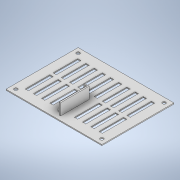
# Autodesk Inventor part: platforma
Saved by Autodesk Inventor 2020.3 (Build 243373000, 373)
## iProperties
Created: 2021-02-15
Part Number: platforma
Material: Ogólny
Document SubType Name: Modeling
Designer: sitar
Density: 1 g/cm^3
Appearance: Domyślna
Author: sitar
Autodesk Inventor part; units mm, degrees
ref_plane "YZ Plane" through (0, 0, 0) normal (1, 0, 0) x (0, 1, 0)
ref_plane "XZ Plane" through (0, 0, 0) normal (0, 1, 0) x (-1, 0, 0)
ref_plane "XY Plane" through (0, 0, 0) normal (0, 0, 1) x (1, 0, 0)
sketch "Szkic1" plane through (0, 0, 0) normal (0, 1, 0) x (-1, 0, 0)
  line L0 (58.5, -44) -> (-58.5, -44)
  line L1 (-58.5, -44) -> (-58.5, 44)
  line L2 (-58.5, 44) -> (58.5, 44)
  line L3 (58.5, 44) -> (58.5, -44)
  line L4 (58.5, -44) -> (-58.5, 44) construction
  line L5 (-58.5, -44) -> (58.5, 44) construction
  point P0 (0, 0)
  dimension "d0" = 117
  dimension "d1" = 88
  constraints: 12 end point, 2 midpoint, 2 parallel, 1 horizontal, 1 perpendicular
  measures "d0" distance of L1.end L2.end
  measures "d1" distance of L0.end L1.end
extrude "Wyciągnięcie proste1" add sketch "Szkic1" along normal blind 1.2
sketch "Szkic2" plane through (0, 1.2, 0) normal (0, 1, 0) x (1, 0, 0)
  line L0 (-52.5, 38) -> (-52.5, 44)
  line L1 (58.5, 44) -> (-58.5, 44) projected
  line L2 (-52.5, 38) -> (-46.5, 38) construction
  line L3 (-52.5, 38) -> (-58.5, 38)
  line L4 (-58.5, 44) -> (-58.5, -44) projected
  line L5 (-52.5, 38) -> (-46.5, 38) construction
  circle A0 centre (-52.5, 38) radius 2
  point P0 (0, 0)
  dimension "d4" = 6
  dimension "d5" = 90
  dimension "d6" = 6
  dimension "d7" = 180
  dimension "d8" = 4
  constraints: 8 end point, 2 equal length, 2 horizontal, 2 perpendicular, 2 point on line, 1 centre point, 1 coincident
  measures "d4" distance of L0.start L0.end
  measures "d5" angle of L2 L0
  measures "d6" distance of L0.start L3.end
  measures "d7" angle of L3 L5
  measures "d8" diameter of A0
extrude "Wyciągnięcie proste2" cut sketch "Szkic2" against normal through all contours L3 A0 L0 | L0 A0 L3
mirror "Odbij1" about plane through (0, 0, 0) normal (0, 0, 1) of "Wyciągnięcie proste2"
mirror "Odbij2" about plane through (0, 0, 0) normal (1, 0, 0) of "Wyciągnięcie proste2", "Odbij1"
sketch "Szkic3" plane through (0, 1.2, 0) normal (0, 1, 0) x (1, 0, 0)
  line L0 (-2.5, -34) -> (-58.5, -34)
  line L1 (-2.5, -34) -> (53.5, -34) construction
  line L2 (-2.5, -34) -> (-2.5, -44)
  line L3 (-2.5, -34) -> (7.5, -34) construction
  line L4 (-58.5, 44) -> (-58.5, -44) projected
  line L5 (-58.5, -44) -> (58.5, -44) projected
  circle A0 centre (-2.5, -34) radius 2
  line L6 (-2.5, -34) -> (-2.5, -12)
  line L7 (-2.5, -34) -> (19.5, -34) construction
  circle A1 centre (-2.5, -12) radius 2
  point P0 (0, 0)
  dimension "d11" = 56
  dimension "d12" = 180
  dimension "d13" = 10
  dimension "d14" = 90
  dimension "d15" = 4
  dimension "d16" = 22
  dimension "d17" = 90
  dimension "d18" = 4
  constraints: 12 end point, 4 horizontal, 3 equal length, 2 centre point, 2 coincident, 2 point on line, 2 vertical
  measures "d11" distance of L0.start L0.end
  measures "d12" angle of L0 L1
  measures "d13" distance of L0.start L2.end
  measures "d14" angle of L2 L3
  measures "d15" diameter of A0
  measures "d16" distance of L6.start L6.end
  measures "d17" angle of L7 L6
  measures "d18" diameter of A1
extrude "Wyciągnięcie proste3" add sketch "Szkic3" along normal blind 2 contours L2 A0 L0 | L6 A0 L2 | L0 A0 L6 | A1
sketch "Szkic4" plane through (-2.5, 3.2, 34) normal (0, 1, 0) x (1, 0, 0)
  circle A0 centre (0, 0) radius 1
  circle A1 centre (0, 22) radius 2 projected
  circle A2 centre (0, 22) radius 1
  point P0 (2.5, 34)
  dimension "d21" = 2
  dimension "d22" = 2
  constraints: 2 centre point, 1 coincident
  measures "d21" diameter of A0
  measures "d22" diameter of A2
extrude "Wyciągnięcie proste4" add sketch "Szkic4" along normal blind 4 contours A0 | A2
sketch "Szkic5" plane through (0, 1.2, 0) normal (0, 1, 0) x (1, 0, 0)
  line L0 (1.5, -4) -> (3.1, -4)
  line L1 (3.1, -4) -> (3.1, -39)
  line L2 (3.1, -39) -> (1.5, -39)
  line L3 (1.5, -39) -> (1.5, -4)
  line L4 (2.3, -39) -> (2.3, -44)
  line L5 (-58.5, -44) -> (58.5, -44) projected
  line L6 (1.5, -15.8672) -> (-58.5, -15.8672)
  line L7 (-58.5, 44) -> (-58.5, -44) projected
  point P0 (0, 0)
  dimension "d25" = 1.6
  dimension "d26" = 35
  dimension "d27" = 5
  dimension "d28" = 60
  constraints: 12 end point, 3 point on line, 2 horizontal, 2 parallel, 2 perpendicular, 1 midpoint
  measures "d25" distance of L1.end L2.end
  measures "d26" distance of L0.end L1.end
  measures "d27" distance of L4.start L4.end
  measures "d28" distance of L6.start L6.end
extrude "Wyciągnięcie proste5" add sketch "Szkic5" along normal blind 14 contours L0 L1 L2 L3
sketch "Szkic6" plane through (0, 1.2, 0) normal (0, 1, 0) x (1, 0, 0)
  line L0 (3.1, -4) -> (1.5, -4) projected
  line L1 (1.5, -4) -> (-2.5, -4)
  line L2 (-2.5, -4) -> (-2.5, -5.2)
  line L3 (-2.5, -5.2) -> (1.5, -5.2)
  line L4 (1.5, -5.2) -> (1.5, -4)
  point P0 (0, 0)
  dimension "d31" = 4
  dimension "d32" = 1.2
  constraints: 8 end point, 2 parallel, 1 horizontal, 1 perpendicular
  measures "d31" distance of L3.end L2.end
  measures "d32" distance of L2.end L1.end
extrude "Wyciągnięcie proste6" add sketch "Szkic6" along normal blind 14
sketch "Szkic7" plane through (0, 1.2, 0) normal (0, 1, 0) x (1, 0, 0)
  line L0 (-47, 32) -> (-43, 32)
  line L1 (-43, 32) -> (-43, 2)
  line L2 (-43, 2) -> (-47, 2)
  line L3 (-47, 2) -> (-47, 32)
  line L4 (-47, 28.7975) -> (-58.5, 28.7975)
  line L5 (-47, 28.7975) -> (-35.5, 28.7975) construction
  line L6 (-58.5, 44) -> (-58.5, -44) projected
  line L7 (-45, 32) -> (-45, 44)
  line L8 (-45, 32) -> (-33, 32) construction
  line L9 (58.5, 44) -> (-58.5, 44) projected
  point P0 (0, 0)
  dimension "d35" = 4
  dimension "d36" = 30
  dimension "d37" = 11.5
  dimension "d38" = 180
  dimension "d39" = 12
  dimension "d40" = 90
  constraints: 16 end point, 3 horizontal, 3 point on line, 2 equal length, 2 parallel, 2 perpendicular, 1 midpoint, 1 vertical
  measures "d35" distance of L1.end L2.end
  measures "d36" distance of L0.end L1.end
  measures "d37" distance of L4.start L4.end
  measures "d38" angle of L4 L5
  measures "d39" distance of L7.start L7.end
  measures "d40" angle of L8 L7
extrude "Wyciągnięcie proste7" cut sketch "Szkic7" against normal through all contours L0 L1 L2 L3
pattern_linear "Szyk prostokątny3" count 10 spacing 10 along (1, 0, 0) of "Wyciągnięcie proste7"
mirror "Odbij5" about plane through (0, 0, 0) normal (0, 0, 1) of "Wyciągnięcie proste7", "Szyk prostokątny3"
sketch "Szkic8" plane through (0, 1.2, 0) normal (0, 1, 0) x (1, 0, 0)
  line L0 (-7, -32) -> (-7, -2) projected
  line L1 (7, -2) -> (-7, -2)
  line L2 (-7, -2) -> (-7, -32)
  line L3 (-7, -32) -> (7, -32)
  line L4 (7, -32) -> (7, -2)
  point P0 (0, 0)
  point P1 (-7, -2)
  constraints: 8 end point, 2 parallel, 1 horizontal, 1 perpendicular
extrude "Wyciągnięcie proste8" add sketch "Szkic8" against normal up to surface (1.2 mm away)
